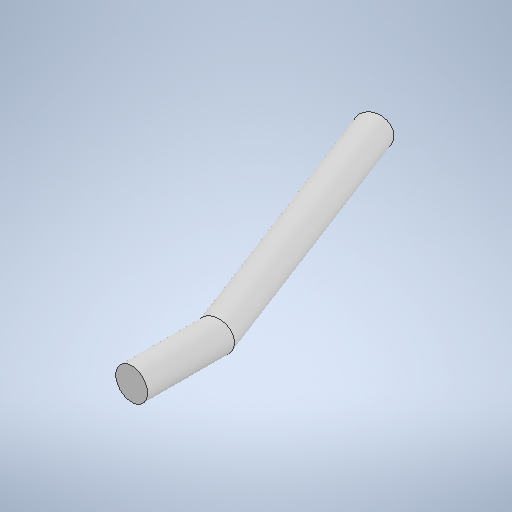
# Autodesk Inventor part: diagonal brace
Saved by Autodesk Inventor 2025 (Build 290162000, 162)
## iProperties
Created: 2024-07-12
Part Number: diagonal brace
Material: 일반
Document SubType Name: Modeling
Designer: unney
Density: 1 g/cm^3
Appearance: 기본값
Author: unney
Autodesk Inventor part; units mm, degrees
ref_plane "YZ Plane" through (0, 0, 0) normal (1, 0, 0) x (0, 1, 0)
ref_plane "XZ Plane" through (0, 0, 0) normal (0, 1, 0) x (-1, 0, 0)
ref_plane "XY Plane" through (0, 0, 0) normal (0, 0, 1) x (1, 0, 0)
sketch "스케치1" plane through (0, 0, 0) normal (0, 0, 1) x (1, 0, 0)
  circle A0 centre (0, 0) radius 8.5
  dimension "d0" = 17
  constraints: 1 centre point, 1 coincident
  measures "d0" diameter of A0
sketch "스케치2" plane through (0, 0, 0) normal (0, 1, 0) x (-1, 0, 0)
  line L0 (0, 0) -> (0, -45)
  line L1 (0, -45) -> (52.6801, -182.2363)
  dimension "d1" = 45
  dimension "d5" = 159
  dimension "d6" = 147
  constraints: 4 end point, 1 vertical
  measures "d1" distance of L0.start L0.end
  measures "d5" angle of L0 L1
  measures "d6" distance of L0.end L1.end
sweep "스윕1" add profiles "스케치1" path "스케치2"
